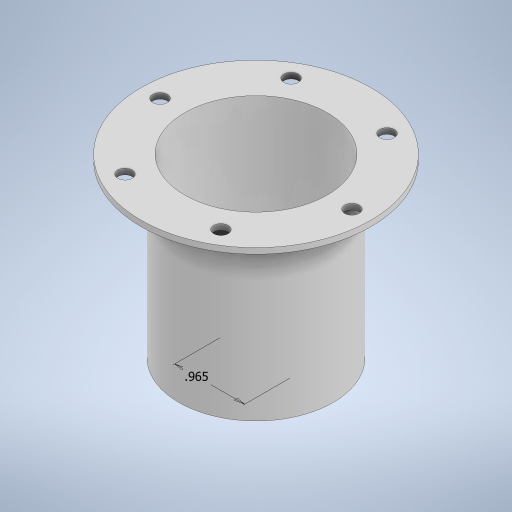
# Autodesk Inventor part: UpstreamVolume
Saved by Autodesk Inventor 2023 (Build 270158000, 158)
## iProperties
Created: 2023-01-27
Part Number: UpstreamVolume
Material: Generic
Document SubType Name: Modeling
Designer: remidm
Density: 1 g/cm^3
Appearance: Default
DistanceBetweenHolesSweep: 0.965 in
Author: remidm
Autodesk Inventor part; units mm, degrees
ref_plane "YZ Plane" through (0, 0, 0) normal (1, 0, 0) x (0, 1, 0)
ref_plane "XZ Plane" through (0, 0, 0) normal (0, 1, 0) x (-1, 0, 0)
ref_plane "XY Plane" through (0, 0, 0) normal (0, 0, 1) x (1, 0, 0)
sketch "Sketch1" plane through (0, 0, 0) normal (0, 0, 1) x (1, 0, 0)
  line L0 (-25, 0) -> (-25, 60)
  line L1 (-25, 60) -> (-40.24, 60)
  line L2 (-40.24, 58) -> (-27, 58)
  line L3 (-27, 58) -> (-27, -2)
  line L4 (-40.24, 58) -> (-40.24, 60)
  line L5 (-25, 0) -> (0, 0)
  line L6 (0, 0) -> (0, -2)
  line L7 (0, -2) -> (-27, -2)
  line L8 (0, -18) -> (0, 73) projected
  dimension "d0" = 2
  dimension "d5" = 2
  dimension "radius" = 25
  dimension "d7" = 2
  dimension "inner_height" = 60
  dimension "d21" = 15.24
  constraints: 16 end point, 3 horizontal, 3 perpendicular
  measures "d0" distance between parallel lines of L1 L2
  measures "d5" distance between parallel lines of L7 L5
  measures "radius" distance from line of L5.end L0
  measures "d7" distance between parallel lines of L0 L3
  measures "inner_height" distance between parallel lines of L5 L1
  measures "d21" distance between parallel lines of L0 L4
revolve "Revolution1" add sketch "Sketch1" angle 360 about axis through (0, -10, 0) along (0, 1, 0)
sketch "Sketch2" plane through (0, 60, 0) normal (0, 1, 0) x (1, 0, 0)
  line L0 (33.62, 0) -> (27, 0)
  circle A0 centre (0, 0) radius 27 projected
  line L1 (33.62, 0) -> (40.24, 0)
  circle A1 centre (0, 0) radius 40.24 projected
  constraints: 4 end point, 2 horizontal alignment, 1 collinear, 1 horizontal, 1 point on line, 2 other
hole "Hole1" at (33.62, 60, 0) direction (0, -1, 0) diameter 5.08 depth 2 tip angle 118
pattern_circular "Circular Pattern1" count 6 over 360 about axis through (0, 59, 0) along (0, 1, 0) of "Hole1"
sketch "Sketch3" plane through (0, -2, 0) normal (0, -1, 0) x (1, 0, 0)
  point P0 (0, 0)
  point P1 (-12.4915, 0)
  point P2 (12.0084, 0)
  dimension "DistanceBetweenHolesSweep" = 24.5
  measures "DistanceBetweenHolesSweep" distance of point (12.008, 0) point (-12.492, 0)
hole "Hole2" at (0, -2, 0) direction (0, 1, 0) diameter 5.08 end through all
hole "Hole3" at (-12.4915, -2, 0) at (12.0084, -2, 0) direction (0, 1, 0) diameter 5 end through all
equation "\"d0\" = thickness"
equation "\"d5\" = thickness"
equation "\"radius\" = 0.5 * SaltDiameter"
equation "\"d7\" = thickness"
equation "\"d21\" = fixation_extension_length"
equation "\"d11\" = fixation_holes_diameter"
equation "\"d22\" = fixation_holes_diameter"
equation "\"d30\" = PenetrationOuterDiameter"
equation "\"thickness\" = crucible_thickness"
equation "\"SaltDiameter\" = 50"
equation "\"fixation_extension_length\" = 15.24"
equation "\"fixation_holes_diameter\" = 5.08"
equation "\"PenetrationOuterDiameter\" = 5"
equation "\"crucible_thickness\" = 2"
body "Solid1"
